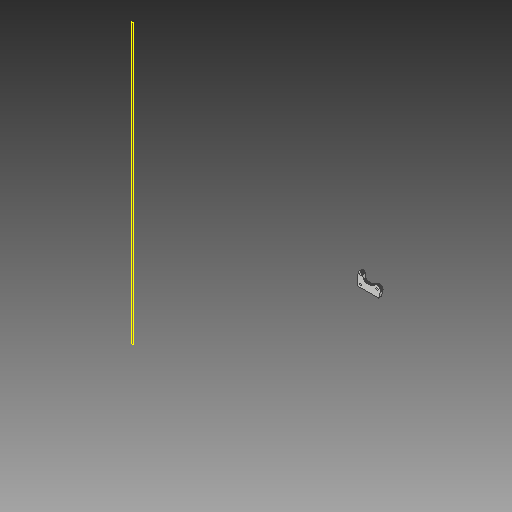
# Autodesk Inventor part: X-Idler
Saved by Autodesk Inventor 2017 (Build 210142000, 142)
## iProperties
Created: 2016-07-20
Part Number: X-Idler
Material: Generic
Document SubType Name: Modeling
Designer: User
Density: 1 g/cm^3
Appearance: Default
Author: User
Autodesk Inventor part; units mm, degrees
ref_plane "YZ Plane" through (0, 0, 0) normal (1, 0, 0) x (0, 1, 0)
ref_plane "XZ Plane" through (0, 0, 0) normal (0, 1, 0) x (-1, 0, 0)
ref_plane "XY Plane" through (0, 0, 0) normal (0, 0, 1) x (1, 0, 0)
ref_plane "Work Plane1" through (12.3, 0, 0) normal (0, 0, 1) x (1, 0, 0)
sketch "Sketch1" plane through (12.3, 0, 0) normal (0, 0, 1) x (1, 0, 0)
  line L0 (532.1042, 356.1222) -> (532.079, 356.3722)
  line L1 (532.079, 356.3722) -> (532.004, 356.6222)
  line L2 (532.004, 356.6222) -> (531.929, 356.8472)
  line L3 (531.929, 356.8472) -> (531.829, 357.0721)
  line L4 (531.829, 357.0721) -> (531.7039, 357.2721)
  line L5 (531.7039, 357.2721) -> (531.5538, 357.4721)
  line L6 (531.5538, 357.4721) -> (531.4038, 357.647)
  line L7 (531.4038, 357.647) -> (531.2287, 357.797)
  line L8 (531.2287, 357.797) -> (531.0287, 357.947)
  line L9 (531.0287, 357.947) -> (530.8288, 358.072)
  line L10 (530.8288, 358.072) -> (530.6037, 358.172)
  line L11 (530.6037, 358.172) -> (530.3788, 358.272)
  line L12 (530.3788, 358.272) -> (530.1288, 358.322)
  line L13 (530.1288, 358.322) -> (529.8788, 358.3721)
  line L14 (529.8788, 358.3721) -> (529.6288, 358.3721)
  line L15 (529.6288, 358.3721) -> (529.3788, 358.3721)
  line L16 (529.3788, 358.3721) -> (529.1288, 358.322)
  line L17 (529.1288, 358.322) -> (528.8788, 358.272)
  line L18 (528.8788, 358.272) -> (528.6538, 358.172)
  line L19 (528.6538, 358.172) -> (528.4288, 358.0719)
  line L20 (528.4288, 358.0719) -> (528.2289, 357.9469)
  line L21 (528.2289, 357.9469) -> (528.0289, 357.7968)
  line L22 (528.0289, 357.7968) -> (527.854, 357.6467)
  line L23 (527.854, 357.6467) -> (527.704, 357.4717)
  line L24 (527.704, 357.4717) -> (527.554, 357.2717)
  line L25 (527.554, 357.2717) -> (527.4289, 357.0717)
  line L26 (527.4289, 357.0717) -> (527.329, 356.8467)
  line L27 (527.329, 356.8467) -> (527.229, 356.6217)
  line L28 (527.229, 356.6217) -> (527.179, 356.3717)
  line L29 (527.179, 356.3717) -> (527.129, 356.1217)
  line L30 (527.129, 356.1217) -> (527.129, 355.8717)
  line L31 (527.129, 355.8717) -> (527.129, 355.6217)
  line L32 (527.129, 355.6217) -> (527.179, 355.3717)
  line L33 (527.179, 355.3717) -> (527.2291, 355.1217)
  line L34 (527.2291, 355.1217) -> (527.3291, 354.8967)
  line L35 (527.3291, 354.8967) -> (527.4291, 354.6718)
  line L36 (527.4291, 354.6718) -> (527.5542, 354.4718)
  line L37 (527.5542, 354.4718) -> (527.7043, 354.2718)
  line L38 (527.7043, 354.2718) -> (527.8543, 354.0969)
  line L39 (527.8543, 354.0969) -> (528.0294, 353.9469)
  line L40 (528.0294, 353.9469) -> (528.2293, 353.7969)
  line L41 (528.2293, 353.7969) -> (528.4293, 353.6719)
  line L42 (528.4293, 353.6719) -> (528.6544, 353.5719)
  line L43 (528.6544, 353.5719) -> (528.8793, 353.4968)
  line L44 (528.8793, 353.4968) -> (529.1293, 353.422)
  line L45 (529.1293, 353.422) -> (529.3794, 353.3972)
  line L46 (529.3794, 353.3972) -> (529.6294, 353.3724)
  line L47 (529.6294, 353.3724) -> (529.8794, 353.3975)
  line L48 (529.8794, 353.3975) -> (530.1294, 353.4227)
  line L49 (530.1294, 353.4227) -> (530.3794, 353.4977)
  line L50 (530.3794, 353.4977) -> (530.6043, 353.5727)
  line L51 (530.6043, 353.5727) -> (530.8293, 353.6728)
  line L52 (530.8293, 353.6728) -> (531.0293, 353.7978)
  line L53 (531.0293, 353.7978) -> (531.2292, 353.9479)
  line L54 (531.2292, 353.9479) -> (531.4042, 354.098)
  line L55 (531.4042, 354.098) -> (531.5542, 354.273)
  line L56 (531.5542, 354.273) -> (531.7049, 354.473)
  line L57 (531.7049, 354.473) -> (531.83, 354.6729)
  line L58 (531.83, 354.6729) -> (531.9299, 354.8979)
  line L59 (531.9299, 354.8979) -> (532.005, 355.1229)
  line L60 (532.005, 355.1229) -> (532.0798, 355.373)
  line L61 (532.0798, 355.373) -> (532.1046, 355.623)
  line L62 (532.1046, 355.623) -> (532.1294, 355.8722)
  line L63 (532.1294, 355.8722) -> (532.1042, 356.1222)
  line L64 (532.1042, 376.8228) -> (532.079, 377.0728)
  line L65 (532.079, 377.0728) -> (532.004, 377.2978)
  line L66 (532.004, 377.2978) -> (531.929, 377.5478)
  line L67 (531.929, 377.5478) -> (531.829, 377.7478)
  line L68 (531.829, 377.7478) -> (531.7039, 377.9477)
  line L69 (531.7039, 377.9477) -> (531.5539, 378.1477)
  line L70 (531.5539, 378.1477) -> (531.4038, 378.3226)
  line L71 (531.4038, 378.3226) -> (531.2288, 378.4976)
  line L72 (531.2288, 378.4976) -> (531.0288, 378.6227)
  line L73 (531.0288, 378.6227) -> (530.8289, 378.7477)
  line L74 (530.8289, 378.7477) -> (530.6039, 378.8728)
  line L75 (530.6039, 378.8728) -> (530.3789, 378.9478)
  line L76 (530.3789, 378.9478) -> (530.1289, 379.0226)
  line L77 (530.1289, 379.0226) -> (529.8789, 379.0475)
  line L78 (529.8789, 379.0475) -> (529.6288, 379.0723)
  line L79 (529.6288, 379.0723) -> (529.3789, 379.0471)
  line L80 (529.3789, 379.0471) -> (529.1289, 379.0219)
  line L81 (529.1289, 379.0219) -> (528.8789, 378.9469)
  line L82 (528.8789, 378.9469) -> (528.6539, 378.8719)
  line L83 (528.6539, 378.8719) -> (528.4289, 378.7468)
  line L84 (528.4289, 378.7468) -> (528.229, 378.6218)
  line L85 (528.229, 378.6218) -> (528.029, 378.4967)
  line L86 (528.029, 378.4967) -> (527.854, 378.3217)
  line L87 (527.854, 378.3217) -> (527.704, 378.1467)
  line L88 (527.704, 378.1467) -> (527.554, 377.9467)
  line L89 (527.554, 377.9467) -> (527.429, 377.7467)
  line L90 (527.429, 377.7467) -> (527.329, 377.5467)
  line L91 (527.329, 377.5467) -> (527.229, 377.2967)
  line L92 (527.229, 377.2967) -> (527.179, 377.0717)
  line L93 (527.179, 377.0717) -> (527.129, 376.8217)
  line L94 (527.129, 376.8217) -> (527.129, 376.5717)
  line L95 (527.129, 376.5717) -> (527.129, 376.2967)
  line L96 (527.129, 376.2967) -> (527.179, 376.0467)
  line L97 (527.179, 376.0467) -> (527.229, 375.8217)
  line L98 (527.229, 375.8217) -> (527.329, 375.5967)
  line L99 (527.329, 375.5967) -> (527.429, 375.3717)
  line L100 (527.429, 375.3717) -> (527.5541, 375.1717)
  line L101 (527.5541, 375.1717) -> (527.7042, 374.9718)
  line L102 (527.7042, 374.9718) -> (527.8543, 374.7968)
  line L103 (527.8543, 374.7968) -> (528.0293, 374.622)
  line L104 (528.0293, 374.622) -> (528.2293, 374.4969)
  line L105 (528.2293, 374.4969) -> (528.4293, 374.3719)
  line L106 (528.4293, 374.3719) -> (528.6543, 374.2468)
  line L107 (528.6543, 374.2468) -> (528.8792, 374.1718)
  line L108 (528.8792, 374.1718) -> (529.1292, 374.1217)
  line L109 (529.1292, 374.1217) -> (529.3792, 374.0717)
  line L110 (529.3792, 374.0717) -> (529.6292, 374.0717)
  line L111 (529.6292, 374.0717) -> (529.8792, 374.0717)
  line L112 (529.8792, 374.0717) -> (530.1292, 374.1217)
  line L113 (530.1292, 374.1217) -> (530.3792, 374.1718)
  line L114 (530.3792, 374.1718) -> (530.6041, 374.2468)
  line L115 (530.6041, 374.2468) -> (530.8291, 374.3719)
  line L116 (530.8291, 374.3719) -> (531.0291, 374.4969)
  line L117 (531.0291, 374.4969) -> (531.229, 374.622)
  line L118 (531.229, 374.622) -> (531.404, 374.797)
  line L119 (531.404, 374.797) -> (531.554, 374.972)
  line L120 (531.554, 374.972) -> (531.704, 375.172)
  line L121 (531.704, 375.172) -> (531.8291, 375.372)
  line L122 (531.8291, 375.372) -> (531.9291, 375.597)
  line L123 (531.9291, 375.597) -> (532.0041, 375.822)
  line L124 (532.0041, 375.822) -> (532.0792, 376.0469)
  line L125 (532.0792, 376.0469) -> (532.104, 376.2969)
  line L126 (532.104, 376.2969) -> (532.1294, 376.5728)
  line L127 (532.1294, 376.5728) -> (532.1042, 376.8228)
  line L128 (569.679, 366.0743) -> (569.6538, 366.3242)
  line L129 (569.6538, 366.3242) -> (569.5788, 366.5742)
  line L130 (569.5788, 366.5742) -> (569.5037, 366.7992)
  line L131 (569.5037, 366.7992) -> (569.4037, 367.0242)
  line L132 (569.4037, 367.0242) -> (569.2787, 367.2241)
  line L133 (569.2787, 367.2241) -> (569.1292, 367.4232)
  line L134 (569.1292, 367.4232) -> (568.9791, 367.5982)
  line L135 (568.9791, 367.5982) -> (568.7791, 367.7482)
  line L136 (568.7791, 367.7482) -> (568.6041, 367.8982)
  line L137 (568.6041, 367.8982) -> (568.4041, 368.0232)
  line L138 (568.4041, 368.0232) -> (568.1791, 368.1232)
  line L139 (568.1791, 368.1232) -> (567.9541, 368.1983)
  line L140 (567.9541, 368.1983) -> (567.7041, 368.2731)
  line L141 (567.7041, 368.2731) -> (567.454, 368.2979)
  line L142 (567.454, 368.2979) -> (567.204, 368.3227)
  line L143 (567.204, 368.3227) -> (566.9541, 368.2975)
  line L144 (566.9541, 368.2975) -> (566.704, 368.2724)
  line L145 (566.704, 368.2724) -> (566.4541, 368.1974)
  line L146 (566.4541, 368.1974) -> (566.2291, 368.1223)
  line L147 (566.2291, 368.1223) -> (566.0041, 368.0223)
  line L148 (566.0041, 368.0223) -> (565.8041, 367.8972)
  line L149 (565.8041, 367.8972) -> (565.6042, 367.7472)
  line L150 (565.6042, 367.7472) -> (565.4291, 367.5966)
  line L151 (565.4291, 367.5966) -> (565.2791, 367.4216)
  line L152 (565.2791, 367.4216) -> (565.129, 367.2217)
  line L153 (565.129, 367.2217) -> (565.004, 367.0217)
  line L154 (565.004, 367.0217) -> (564.904, 366.7967)
  line L155 (564.904, 366.7967) -> (564.8041, 366.5717)
  line L156 (564.8041, 366.5717) -> (564.754, 366.3217)
  line L157 (564.754, 366.3217) -> (564.704, 366.0717)
  line L158 (564.704, 366.0717) -> (564.704, 365.8217)
  line L159 (564.704, 365.8217) -> (564.704, 365.5717)
  line L160 (564.704, 365.5717) -> (564.754, 365.3217)
  line L161 (564.754, 365.3217) -> (564.8041, 365.0717)
  line L162 (564.8041, 365.0717) -> (564.9041, 364.8467)
  line L163 (564.9041, 364.8467) -> (565.0041, 364.6217)
  line L164 (565.0041, 364.6217) -> (565.1292, 364.4218)
  line L165 (565.1292, 364.4218) -> (565.2793, 364.2218)
  line L166 (565.2793, 364.2218) -> (565.4294, 364.0469)
  line L167 (565.4294, 364.0469) -> (565.6044, 363.8969)
  line L168 (565.6044, 363.8969) -> (565.804, 363.7464)
  line L169 (565.804, 363.7464) -> (566.004, 363.6214)
  line L170 (566.004, 363.6214) -> (566.229, 363.5214)
  line L171 (566.229, 363.5214) -> (566.454, 363.4214)
  line L172 (566.454, 363.4214) -> (566.704, 363.3715)
  line L173 (566.704, 363.3715) -> (566.954, 363.3215)
  line L174 (566.954, 363.3215) -> (567.204, 363.3215)
  line L175 (567.204, 363.3215) -> (567.454, 363.3215)
  line L176 (567.454, 363.3215) -> (567.704, 363.3715)
  line L177 (567.704, 363.3715) -> (567.9541, 363.4216)
  line L178 (567.9541, 363.4216) -> (568.1792, 363.5216)
  line L179 (568.1792, 363.5216) -> (568.4041, 363.6217)
  line L180 (568.4041, 363.6217) -> (568.6041, 363.7467)
  line L181 (568.6041, 363.7467) -> (568.779, 363.8968)
  line L182 (568.779, 363.8968) -> (568.979, 364.0469)
  line L183 (568.979, 364.0469) -> (569.129, 364.2219)
  line L184 (569.129, 364.2219) -> (569.2795, 364.4223)
  line L185 (569.2795, 364.4223) -> (569.4045, 364.6223)
  line L186 (569.4045, 364.6223) -> (569.5045, 364.8473)
  line L187 (569.5045, 364.8473) -> (569.5796, 365.0723)
  line L188 (569.5796, 365.0723) -> (569.6547, 365.3236)
  line L189 (569.6547, 365.3236) -> (569.6796, 365.5735)
  line L190 (569.6796, 365.5735) -> (569.7043, 365.8226)
  line L191 (569.7043, 365.8226) -> (569.679, 366.0743)
  line L192 (574.9801, 366.7498) -> (574.9051, 367.3498)
  line L193 (574.9051, 367.3498) -> (574.7549, 367.9497)
  line L194 (574.7549, 367.9497) -> (574.5548, 368.5497)
  line L195 (574.5548, 368.5497) -> (574.3299, 369.0998)
  line L196 (574.3299, 369.0998) -> (574.055, 369.6498)
  line L197 (574.055, 369.6498) -> (573.7298, 370.1747)
  line L198 (573.7298, 370.1747) -> (573.3546, 370.6745)
  line L199 (573.3546, 370.6745) -> (572.9545, 371.1494)
  line L200 (572.9545, 371.1494) -> (572.5295, 371.5744)
  line L201 (572.5295, 371.5744) -> (572.0544, 371.9744)
  line L202 (572.0544, 371.9744) -> (571.5545, 372.3494)
  line L203 (571.5545, 372.3494) -> (571.0294, 372.6743)
  line L204 (571.0294, 372.6743) -> (570.4794, 372.9492)
  line L205 (570.4794, 372.9492) -> (569.9044, 373.1743)
  line L206 (569.9044, 373.1743) -> (569.3294, 373.3743)
  line L207 (569.3294, 373.3743) -> (568.7294, 373.5243)
  line L208 (568.7294, 373.5243) -> (568.1294, 373.6243)
  line L209 (568.1294, 373.6243) -> (567.5044, 373.6493)
  line L210 (567.5044, 373.6493) -> (566.8794, 373.6493)
  line L211 (566.8794, 373.6493) -> (566.2794, 373.6242)
  line L212 (566.2794, 373.6242) -> (565.6794, 373.5241)
  line L213 (565.6794, 373.5241) -> (565.0794, 373.374)
  line L214 (565.0794, 373.374) -> (564.4795, 373.1739)
  line L215 (564.4795, 373.1739) -> (563.9045, 372.9489)
  line L216 (563.9045, 372.9489) -> (563.3545, 372.6739)
  line L217 (563.3545, 372.6739) -> (562.8296, 372.3487)
  line L218 (562.8296, 372.3487) -> (562.3297, 371.9736)
  line L219 (562.3297, 371.9736) -> (561.8548, 371.5734)
  line L220 (561.8548, 371.5734) -> (561.43, 371.1233)
  line L221 (561.43, 371.1233) -> (561.0301, 370.6732)
  line L222 (561.0301, 370.6732) -> (560.6553, 370.148)
  line L223 (560.6553, 370.148) -> (559.8804, 369.5979)
  line L224 (559.8804, 369.5979) -> (559.1056, 369.0976)
  line L225 (559.1056, 369.0976) -> (558.3057, 368.5974)
  line L226 (558.3057, 368.5974) -> (557.4807, 368.1474)
  line L227 (557.4807, 368.1474) -> (556.6306, 367.7225)
  line L228 (556.6306, 367.7225) -> (555.7557, 367.3475)
  line L229 (555.7557, 367.3475) -> (554.8807, 366.9975)
  line L230 (554.8807, 366.9975) -> (554.0057, 366.6725)
  line L231 (554.0057, 366.6725) -> (553.1057, 366.3975)
  line L232 (553.1057, 366.3975) -> (552.1807, 366.1475)
  line L233 (552.1807, 366.1475) -> (551.2557, 365.9225)
  line L234 (551.2557, 365.9225) -> (550.3306, 365.7475)
  line L235 (550.3306, 365.7475) -> (549.4057, 365.6225)
  line L236 (549.4057, 365.6225) -> (548.4807, 365.5225)
  line L237 (548.4807, 365.5225) -> (547.5307, 365.4475)
  line L238 (547.5307, 365.4475) -> (546.5807, 365.4225)
  line L239 (546.5807, 365.4225) -> (545.8056, 365.4225)
  line L240 (545.8056, 365.4225) -> (545.0307, 365.4474)
  line L241 (545.0307, 365.4474) -> (544.2807, 365.4974)
  line L242 (544.2807, 365.4974) -> (543.5057, 365.5975)
  line L243 (543.5057, 365.5975) -> (542.8307, 365.6225)
  line L244 (542.8307, 365.6225) -> (542.1807, 365.7225)
  line L245 (542.1807, 365.7225) -> (541.5306, 365.8475)
  line L246 (541.5306, 365.8475) -> (540.8807, 366.0475)
  line L247 (540.8807, 366.0475) -> (540.2557, 366.2976)
  line L248 (540.2557, 366.2976) -> (539.6557, 366.5725)
  line L249 (539.6557, 366.5725) -> (539.0806, 366.9224)
  line L250 (539.0806, 366.9224) -> (538.5305, 367.2974)
  line L251 (538.5305, 367.2974) -> (538.0055, 367.7223)
  line L252 (538.0055, 367.7223) -> (537.5305, 368.1722)
  line L253 (537.5305, 368.1722) -> (537.0804, 368.6722)
  line L254 (537.0804, 368.6722) -> (536.6803, 369.2221)
  line L255 (536.6803, 369.2221) -> (536.3802, 369.6721)
  line L256 (536.3802, 369.6721) -> (536.1052, 370.147)
  line L257 (536.1052, 370.147) -> (534.5542, 378.3219)
  line L258 (534.5542, 378.3219) -> (534.4791, 378.7218)
  line L259 (534.4791, 378.7218) -> (534.3791, 379.0968)
  line L260 (534.3791, 379.0968) -> (534.2541, 379.4718)
  line L261 (534.2541, 379.4718) -> (534.0791, 379.8218)
  line L262 (534.0791, 379.8218) -> (533.9041, 380.1719)
  line L263 (533.9041, 380.1719) -> (533.6791, 380.4968)
  line L264 (533.6791, 380.4968) -> (533.4291, 380.7969)
  line L265 (533.4291, 380.7969) -> (533.1791, 381.0969)
  line L266 (533.1791, 381.0969) -> (532.8791, 381.3469)
  line L267 (532.8791, 381.3469) -> (532.5792, 381.5969)
  line L268 (532.5792, 381.5969) -> (532.2541, 381.8219)
  line L269 (532.2541, 381.8219) -> (531.9041, 381.9968)
  line L270 (531.9041, 381.9968) -> (531.5541, 382.1718)
  line L271 (531.5541, 382.1718) -> (531.1791, 382.3218)
  line L272 (531.1791, 382.3218) -> (530.8041, 382.4218)
  line L273 (530.8041, 382.4218) -> (530.4291, 382.4969)
  line L274 (530.4291, 382.4969) -> (530.0291, 382.5468)
  line L275 (530.0291, 382.5468) -> (529.6541, 382.5718)
  line L276 (529.6541, 382.5718) -> (529.2541, 382.5467)
  line L277 (529.2541, 382.5467) -> (528.8791, 382.4967)
  line L278 (528.8791, 382.4967) -> (528.4792, 382.4217)
  line L279 (528.4792, 382.4217) -> (528.1041, 382.3216)
  line L280 (528.1041, 382.3216) -> (527.7291, 382.1966)
  line L281 (527.7291, 382.1966) -> (527.3792, 382.0216)
  line L282 (527.3792, 382.0216) -> (527.0291, 381.8466)
  line L283 (527.0291, 381.8466) -> (526.7041, 381.6217)
  line L284 (526.7041, 381.6217) -> (526.4041, 381.3717)
  line L285 (526.4041, 381.3717) -> (526.1041, 381.1217)
  line L286 (526.1041, 381.1217) -> (525.8541, 380.8217)
  line L287 (525.8541, 380.8217) -> (525.6041, 380.5217)
  line L288 (525.6041, 380.5217) -> (525.3791, 380.1967)
  line L289 (525.3791, 380.1967) -> (525.1791, 379.8466)
  line L290 (525.1791, 379.8466) -> (525.0291, 379.4967)
  line L291 (525.0291, 379.4967) -> (524.8791, 379.1217)
  line L292 (524.8791, 379.1217) -> (524.779, 378.7467)
  line L293 (524.779, 378.7467) -> (524.704, 378.3717)
  line L294 (524.704, 378.3717) -> (524.654, 377.9717)
  line L295 (524.654, 377.9717) -> (524.629, 377.5717)
  line L296 (524.629, 377.5717) -> (522.954, 368.6217)
  line L297 (522.954, 368.6217) -> (522.954, 349.8812)
  line L298 (522.954, 349.8812) -> (570.8611, 349.8812)
  line L299 (570.8611, 349.8812) -> (574.7613, 363.7062)
  line L300 (574.7613, 363.7062) -> (574.9113, 364.3062)
  line L301 (574.9113, 364.3062) -> (574.9863, 364.9062)
  line L302 (574.9863, 364.9062) -> (575.0302, 365.5316)
  line L303 (575.0302, 365.5316) -> (575.0302, 366.1248)
  line L304 (575.0302, 366.1248) -> (574.9801, 366.7498)
  point P0 (-12.3, 0)
  constraints: 610 end point, 99 parallel, 94 perpendicular, 11 collinear
extrude "Extrusion1" add sketch "Sketch1" along normal blind 6
sketch "Sketch2" plane through (12.3, 0, 6) normal (0, 0, 1) x (1, 0, 0)
  line L0 (529.3794, 353.3972) -> (529.6294, 353.3724) projected
  line L1 (529.6294, 353.3724) -> (529.6288, 358.3721)
  line L2 (529.8788, 358.3721) -> (529.3788, 358.3721) projected
  line L3 (529.8792, 374.0717) -> (529.3792, 374.0717) projected
  line L4 (529.6288, 379.0723) -> (529.3789, 379.0471) projected
  line L5 (529.6292, 374.0717) -> (529.6288, 379.0723)
  line L6 (566.9541, 368.2975) -> (567.204, 368.3227) projected
  line L7 (567.204, 368.3227) -> (567.204, 363.3215)
  line L8 (567.454, 363.3215) -> (566.954, 363.3215) projected
  point P0 (-12.3, 0)
  point P1 (567.204, 365.8221)
  point P2 (529.6291, 355.8722)
  point P3 (529.629, 376.572)
  constraints: 6 end point, 6 midpoint
hole "Hole1" at (579.504, 365.8221, 6) at (541.9291, 355.8722, 6) at (541.929, 376.572, 6) direction (0, 0, -1) diameter 5.2 end through all
body "Solid1"
